Autodesk Fusion 360 part; units mm, degrees
(part 3 of 10)
  line L1783 (-29.0015, -12.4722) -> (-29.0035, -12.4576)
  line L1784 (-29.0035, -12.4576) -> (-28.9989, -12.4287)
  line L1785 (-28.9989, -12.4287) -> (-28.9835, -12.4038)
  line L1786 (-28.9835, -12.4038) -> (-28.9598, -12.3866)
  line L1787 (-28.9598, -12.3866) -> (-28.9314, -12.3799)
  line L1788 (-28.9314, -12.3799) -> (-28.9025, -12.3845)
  line L1789 (-28.9025, -12.3845) -> (-28.8776, -12.3998)
  line L1790 (-28.8776, -12.3998) -> (-28.8604, -12.4235)
  line L1791 (-28.8604, -12.4235) -> (-28.8556, -12.4374)
  line L1792 (-28.8556, -12.4374) -> (-28.6864, -13.1483)
  line L1793 (-28.6864, -13.1483) -> (-28.5725, -12.7212)
  line L1794 (-28.5725, -12.7212) -> (-28.5712, -12.7178)
  line L1795 (-28.5712, -12.7178) -> (-28.571, -12.7163)
  line L1796 (-28.571, -12.7163) -> (-28.57, -12.7146)
  line L1797 (-28.57, -12.7146) -> (-28.5673, -12.7074)
  line L1798 (-28.5673, -12.7074) -> (-28.5613, -12.6996)
  line L1799 (-28.5613, -12.6996) -> (-28.5563, -12.691)
  line L1800 (-28.5563, -12.691) -> (-28.5525, -12.6881)
  line L1801 (-28.5525, -12.6881) -> (-28.5495, -12.6842)
  line L1802 (-28.5495, -12.6842) -> (-28.541, -12.6792)
  line L1803 (-28.541, -12.6792) -> (-28.5331, -12.6732)
  line L1804 (-28.5331, -12.6732) -> (-28.5284, -12.672)
  line L1805 (-28.5284, -12.672) -> (-28.5242, -12.6695)
  line L1806 (-28.5242, -12.6695) -> (-28.5144, -12.6682)
  line L1807 (-28.5144, -12.6682) -> (-28.5048, -12.6657)
  line L1808 (-28.5048, -12.6657) -> (-28.5, -12.6663)
  line L1809 (-28.5, -12.6663) -> (-28.4952, -12.6657)
  line L1810 (-28.4952, -12.6657) -> (-28.4856, -12.6682)
  line L1811 (-28.4856, -12.6682) -> (-28.4758, -12.6695)
  line L1812 (-28.4758, -12.6695) -> (-28.4716, -12.672)
  line L1813 (-28.4716, -12.672) -> (-28.4669, -12.6732)
  line L1814 (-28.4669, -12.6732) -> (-28.459, -12.6792)
  line L1815 (-28.459, -12.6792) -> (-28.4505, -12.6842)
  line L1816 (-28.4505, -12.6842) -> (-28.4475, -12.6881)
  line L1817 (-28.4475, -12.6881) -> (-28.4437, -12.691)
  line L1818 (-28.4437, -12.691) -> (-28.4387, -12.6996)
  line L1819 (-28.4387, -12.6996) -> (-28.4327, -12.7074)
  line L1820 (-28.4327, -12.7074) -> (-28.43, -12.7146)
  line L1821 (-28.43, -12.7146) -> (-28.429, -12.7163)
  line L1822 (-28.429, -12.7163) -> (-28.4288, -12.7178)
  line L1823 (-28.4288, -12.7178) -> (-28.4275, -12.7212)
  line L1824 (-28.4275, -12.7212) -> (-28.3136, -13.1483)
  line L1825 (-28.3136, -13.1483) -> (-28.1444, -12.4374)
  line L1826 (-28.1444, -12.4374) -> (-28.1396, -12.4235)
  line L1827 (-28.1396, -12.4235) -> (-28.1224, -12.3998)
  line L1828 (-28.1224, -12.3998) -> (-28.0975, -12.3845)
  line L1829 (-28.0975, -12.3845) -> (-28.0686, -12.3799)
  line L1830 (-28.0686, -12.3799) -> (-28.0402, -12.3867)
  line L1831 (-19.702, -11.3796) -> (-19.6696, -11.412)
  line L1832 (-19.6696, -11.412) -> (-19.665, -11.435)
  line L1833 (-19.665, -11.435) -> (-19.665, -25.405)
  line L1834 (-19.665, -25.405) -> (-19.6696, -25.428)
  line L1835 (-19.6696, -25.428) -> (-19.702, -25.4604)
  line L1836 (-19.702, -25.4604) -> (-19.725, -25.465)
  line L1837 (-19.725, -25.465) -> (-33.695, -25.465)
  line L1838 (-33.695, -25.465) -> (-33.718, -25.4604)
  line L1839 (-33.718, -25.4604) -> (-33.7504, -25.428)
  line L1840 (-33.7504, -25.428) -> (-33.755, -25.405)
  line L1841 (-33.755, -25.405) -> (-33.755, -11.435)
  line L1842 (-33.755, -11.435) -> (-33.7504, -11.412)
  line L1843 (-33.7504, -11.412) -> (-33.718, -11.3796)
  line L1844 (-33.718, -11.3796) -> (-33.695, -11.375)
  line L1845 (-33.695, -11.375) -> (-19.725, -11.375)
  line L1846 (-19.725, -11.375) -> (-19.702, -11.3796)
  line L1847 (-33.635, -11.495) -> (-33.635, -25.345)
  line L1848 (-33.635, -25.345) -> (-19.785, -25.345)
  line L1849 (-19.785, -25.345) -> (-19.785, -11.495)
  line L1850 (-19.785, -11.495) -> (-33.635, -11.495)
  line L1851 (-14.3974, -12.3805) -> (-14.3954, -12.3804)
  line L1852 (-14.3954, -12.3804) -> (-14.3928, -12.381)
  line L1853 (-14.3928, -12.381) -> (-14.3901, -12.3813)
  line L1854 (-14.3901, -12.3813) -> (-14.3883, -12.382)
  line L1855 (-14.3883, -12.382) -> (-14.381, -12.3837)
  line L1856 (-14.381, -12.3837) -> (-14.2382, -12.4313)
  line L1857 (-14.2382, -12.4313) -> (-14.2248, -12.4373)
  line L1858 (-14.2248, -12.4373) -> (-14.2027, -12.4565)
  line L1859 (-14.2027, -12.4565) -> (-14.1896, -12.4826)
  line L1860 (-14.1896, -12.4826) -> (-14.1875, -12.5118)
  line L1861 (-14.1875, -12.5118) -> (-14.1967, -12.5396)
  line L1862 (-14.1967, -12.5396) -> (-14.2159, -12.5617)
  line L1863 (-14.2159, -12.5617) -> (-14.2421, -12.5748)
  line L1864 (-14.2421, -12.5748) -> (-14.2713, -12.5768)
  line L1865 (-14.2713, -12.5768) -> (-14.2856, -12.5736)
  line L1866 (-14.2856, -12.5736) -> (-14.4169, -12.5298)
  line L1867 (-14.4169, -12.5298) -> (-14.6252, -12.5298)
  line L1868 (-14.6252, -12.5298) -> (-14.6937, -12.5641)
  line L1869 (-14.6937, -12.5641) -> (-14.7241, -12.5945)
  line L1870 (-14.7241, -12.5945) -> (-14.7583, -12.663)
  line L1871 (-14.7583, -12.663) -> (-14.7583, -12.7228)
  line L1872 (-14.7583, -12.7228) -> (-14.7241, -12.7913)
  line L1873 (-14.7241, -12.7913) -> (-14.6937, -12.8218)
  line L1874 (-14.6937, -12.8218) -> (-14.6167, -12.8602)
  line L1875 (-14.6167, -12.8602) -> (-14.4342, -12.9059)
  line L1876 (-14.4342, -12.9059) -> (-14.4331, -12.9063)
  line L1877 (-14.4331, -12.9063) -> (-14.4326, -12.9063)
  line L1878 (-14.4326, -12.9063) -> (-14.4265, -12.9086)
  line L1879 (-14.4265, -12.9086) -> (-14.4203, -12.9108)
  line L1880 (-14.4203, -12.9108) -> (-14.4199, -12.9111)
  line L1881 (-14.4199, -12.9111) -> (-14.4188, -12.9115)
  line L1882 (-14.4188, -12.9115) -> (-14.3236, -12.9592)
  line L1883 (-14.3236, -12.9592) -> (-14.3173, -12.9631)
  line L1884 (-14.3173, -12.9631) -> (-14.3155, -12.9639)
  line L1885 (-14.3155, -12.9639) -> (-14.3134, -12.9656)
  line L1886 (-14.3134, -12.9656) -> (-14.3112, -12.967)
  line L1887 (-14.3112, -12.967) -> (-14.3099, -12.9685)
  line L1888 (-14.3099, -12.9685) -> (-14.3041, -12.9732)
  line L1889 (-14.3041, -12.9732) -> (-14.2565, -13.0208)
  line L1890 (-14.2565, -13.0208) -> (-14.2518, -13.0266)
  line L1891 (-14.2518, -13.0266) -> (-14.2503, -13.0279)
  line L1892 (-14.2503, -13.0279) -> (-14.2489, -13.0301)
  line L1893 (-14.2489, -13.0301) -> (-14.2472, -13.0322)
  line L1894 (-14.2472, -13.0322) -> (-14.2464, -13.034)
  line L1895 (-14.2464, -13.034) -> (-14.2424, -13.0403)
  line L1896 (-14.2424, -13.0403) -> (-14.1948, -13.1356)
  line L1897 (-14.1948, -13.1356) -> (-14.1896, -13.1493)
  line L1898 (-14.1896, -13.1493) -> (-14.1894, -13.152)
  line L1899 (-14.1894, -13.152) -> (-14.1883, -13.1545)
  line L1900 (-14.1883, -13.1545) -> (-14.1869, -13.1691)
  line L1901 (-14.1869, -13.1691) -> (-14.1869, -13.2643)
  line L1902 (-14.1869, -13.2643) -> (-14.1883, -13.279)
  line L1903 (-14.1883, -13.279) -> (-14.1894, -13.2815)
  line L1904 (-14.1894, -13.2815) -> (-14.1896, -13.2842)
  line L1905 (-14.1896, -13.2842) -> (-14.1948, -13.2979)
  line L1906 (-14.1948, -13.2979) -> (-14.2424, -13.3931)
  line L1907 (-14.2424, -13.3931) -> (-14.2464, -13.3994)
  line L1908 (-14.2464, -13.3994) -> (-14.2472, -13.4012)
  line L1909 (-14.2472, -13.4012) -> (-14.2489, -13.4033)
  line L1910 (-14.2489, -13.4033) -> (-14.2503, -13.4056)
  line L1911 (-14.2503, -13.4056) -> (-14.2518, -13.4069)
  line L1912 (-14.2518, -13.4069) -> (-14.2565, -13.4126)
  line L1913 (-14.2565, -13.4126) -> (-14.3041, -13.4602)
  line L1914 (-14.3041, -13.4602) -> (-14.3099, -13.4649)
  line L1915 (-14.3099, -13.4649) -> (-14.3112, -13.4665)
  line L1916 (-14.3112, -13.4665) -> (-14.3134, -13.4679)
  line L1917 (-14.3134, -13.4679) -> (-14.3155, -13.4696)
  line L1918 (-14.3155, -13.4696) -> (-14.3173, -13.4703)
  line L1919 (-14.3173, -13.4703) -> (-14.3236, -13.4743)
  line L1920 (-14.3236, -13.4743) -> (-14.4188, -13.5219)
  line L1921 (-14.4188, -13.5219) -> (-14.4326, -13.5272)
  line L1922 (-14.4326, -13.5272) -> (-14.4353, -13.5273)
  line L1923 (-14.4353, -13.5273) -> (-14.4377, -13.5284)
  line L1924 (-14.4377, -13.5284) -> (-14.4524, -13.5298)
  line L1925 (-14.4524, -13.5298) -> (-14.6905, -13.5298)
  line L1926 (-14.6905, -13.5298) -> (-14.6979, -13.5291)
  line L1927 (-14.6979, -13.5291) -> (-14.6999, -13.5292)
  line L1928 (-14.6999, -13.5292) -> (-14.7025, -13.5286)
  line L1929 (-14.7025, -13.5286) -> (-14.7051, -13.5284)
  line L1930 (-14.7051, -13.5284) -> (-14.7069, -13.5276)
  line L1931 (-14.7069, -13.5276) -> (-14.7142, -13.526)
  line L1932 (-14.7142, -13.526) -> (-14.857, -13.4784)
  line L1933 (-14.857, -13.4784) -> (-14.8705, -13.4724)
  line L1934 (-14.8705, -13.4724) -> (-14.8926, -13.4532)
  line L1935 (-14.8926, -13.4532) -> (-14.9057, -13.427)
  line L1936 (-14.9057, -13.427) -> (-14.9077, -13.3978)
  line L1937 (-14.9077, -13.3978) -> (-14.8985, -13.3701)
  line L1938 (-14.8985, -13.3701) -> (-14.8793, -13.3479)
  line L1939 (-14.8793, -13.3479) -> (-14.8531, -13.3349)
  line L1940 (-14.8531, -13.3349) -> (-14.824, -13.3328)
  line L1941 (-14.824, -13.3328) -> (-14.8096, -13.336)
  line L1942 (-14.8096, -13.336) -> (-14.6783, -13.3798)
  line L1943 (-14.6783, -13.3798) -> (-14.4701, -13.3798)
  line L1944 (-14.4701, -13.3798) -> (-14.4016, -13.3456)
  line L1945 (-14.4016, -13.3456) -> (-14.3712, -13.3152)
  line L1946 (-14.3712, -13.3152) -> (-14.3369, -13.2466)
  line L1947 (-14.3369, -13.2466) -> (-14.3369, -13.1868)
  line L1948 (-14.3369, -13.1868) -> (-14.3712, -13.1183)
  line L1949 (-14.3712, -13.1183) -> (-14.4016, -13.0879)
  line L1950 (-14.4016, -13.0879) -> (-14.4786, -13.0494)
  line L1951 (-14.4786, -13.0494) -> (-14.661, -13.0038)
  line L1952 (-14.661, -13.0038) -> (-14.6621, -13.0034)
  line L1953 (-14.6621, -13.0034) -> (-14.6627, -13.0033)
  line L1954 (-14.6627, -13.0033) -> (-14.6688, -13.001)
  line L1955 (-14.6688, -13.001) -> (-14.6749, -12.9988)
  line L1956 (-14.6749, -12.9988) -> (-14.6753, -12.9985)
  line L1957 (-14.6753, -12.9985) -> (-14.6764, -12.9981)
  line L1958 (-14.6764, -12.9981) -> (-14.7716, -12.9505)
  line L1959 (-14.7716, -12.9505) -> (-14.7779, -12.9465)
  line L1960 (-14.7779, -12.9465) -> (-14.7798, -12.9458)
  line L1961 (-14.7798, -12.9458) -> (-14.7818, -12.9441)
  line L1962 (-14.7818, -12.9441) -> (-14.7841, -12.9426)
  line L1963 (-14.7841, -12.9426) -> (-14.7854, -12.9411)
  line L1964 (-14.7854, -12.9411) -> (-14.7911, -12.9364)
  line L1965 (-14.7911, -12.9364) -> (-14.8387, -12.8888)
  line L1966 (-14.8387, -12.8888) -> (-14.8435, -12.8831)
  line L1967 (-14.8435, -12.8831) -> (-14.845, -12.8818)
  line L1968 (-14.845, -12.8818) -> (-14.8464, -12.8795)
  line L1969 (-14.8464, -12.8795) -> (-14.8481, -12.8774)
  line L1970 (-14.8481, -12.8774) -> (-14.8488, -12.8756)
  line L1971 (-14.8488, -12.8756) -> (-14.8528, -12.8693)
  line L1972 (-14.8528, -12.8693) -> (-14.9004, -12.7741)
  line L1973 (-14.9004, -12.7741) -> (-14.9057, -12.7603)
  line L1974 (-14.9057, -12.7603) -> (-14.9059, -12.7577)
  line L1975 (-14.9059, -12.7577) -> (-14.9069, -12.7552)
  line L1976 (-14.9069, -12.7552) -> (-14.9083, -12.7405)
  line L1977 (-14.9083, -12.7405) -> (-14.9083, -12.6453)
  line L1978 (-14.9083, -12.6453) -> (-14.9069, -12.6307)
  line L1979 (-14.9069, -12.6307) -> (-14.9059, -12.6282)
  line L1980 (-14.9059, -12.6282) -> (-14.9057, -12.6255)
  line L1981 (-14.9057, -12.6255) -> (-14.9004, -12.6118)
  line L1982 (-14.9004, -12.6118) -> (-14.8528, -12.5165)
  line L1983 (-14.8528, -12.5165) -> (-14.8488, -12.5102)
  line L1984 (-14.8488, -12.5102) -> (-14.8481, -12.5084)
  line L1985 (-14.8481, -12.5084) -> (-14.8464, -12.5063)
  line L1986 (-14.8464, -12.5063) -> (-14.845, -12.5041)
  line L1987 (-14.845, -12.5041) -> (-14.8435, -12.5028)
  line L1988 (-14.8435, -12.5028) -> (-14.8387, -12.497)
  line L1989 (-14.8387, -12.497) -> (-14.7911, -12.4494)
  line L1990 (-14.7911, -12.4494) -> (-14.7854, -12.4447)
  line L1991 (-14.7854, -12.4447) -> (-14.7841, -12.4432)
  line L1992 (-14.7841, -12.4432) -> (-14.7818, -12.4418)
  line L1993 (-14.7818, -12.4418) -> (-14.7798, -12.4401)
  line L1994 (-14.7798, -12.4401) -> (-14.7779, -12.4393)
  line L1995 (-14.7779, -12.4393) -> (-14.7716, -12.4354)
  line L1996 (-14.7716, -12.4354) -> (-14.6764, -12.3877)
  line L1997 (-14.6764, -12.3877) -> (-14.6627, -12.3825)
  line L1998 (-14.6627, -12.3825) -> (-14.66, -12.3823)
  line L1999 (-14.66, -12.3823) -> (-14.6575, -12.3813)
  line L2000 (-14.6575, -12.3813) -> (-14.6429, -12.3798)
  line L2001 (-14.6429, -12.3798) -> (-14.4048, -12.3798)
  line L2002 (-14.4048, -12.3798) -> (-14.3974, -12.3805)
  line L2003 (-12.2473, -12.3813) -> (-12.2202, -12.3925)
  line L2004 (-12.2202, -12.3925) -> (-12.1995, -12.4132)
  line L2005 (-12.1995, -12.4132) -> (-12.1883, -12.4402)
  line L2006 (-12.1883, -12.4402) -> (-12.1883, -12.4695)
  line L2007 (-12.1883, -12.4695) -> (-12.1995, -12.4965)
  line L2008 (-12.1995, -12.4965) -> (-12.2202, -12.5172)
  line L2009 (-12.2202, -12.5172) -> (-12.2473, -12.5284)
  line L2010 (-12.2473, -12.5284) -> (-12.2619, -12.5298)
  line L2011 (-12.2619, -12.5298) -> (-12.4347, -12.5298)
  line L2012 (-12.4347, -12.5298) -> (-12.5032, -12.5641)
  line L2013 (-12.5032, -12.5641) -> (-12.537, -12.5978)
  line L2014 (-12.537, -12.5978) -> (-12.6209, -12.7237)
  line L2015 (-12.6209, -12.7237) -> (-12.6394, -12.7978)
  line L2016 (-12.6394, -12.7978) -> (-12.5812, -12.7687)
  line L2017 (-12.5812, -12.7687) -> (-12.5674, -12.7634)
  line L2018 (-12.5674, -12.7634) -> (-12.5647, -12.7632)
  line L2019 (-12.5647, -12.7632) -> (-12.5623, -12.7622)
  line L2020 (-12.5623, -12.7622) -> (-12.5476, -12.7608)
  line L2021 (-12.5476, -12.7608) -> (-12.3571, -12.7608)
  line L2022 (-12.3571, -12.7608) -> (-12.3425, -12.7622)
  line L2023 (-12.3425, -12.7622) -> (-12.34, -12.7632)
  line L2024 (-12.34, -12.7632) -> (-12.3373, -12.7634)
  line L2025 (-12.3373, -12.7634) -> (-12.3236, -12.7687)
  line L2026 (-12.3236, -12.7687) -> (-12.2284, -12.8163)
  line L2027 (-12.2284, -12.8163) -> (-12.2221, -12.8203)
  line L2028 (-12.2221, -12.8203) -> (-12.2202, -12.821)
  line L2029 (-12.2202, -12.821) -> (-12.2182, -12.8227)
  line L2030 (-12.2182, -12.8227) -> (-12.2159, -12.8241)
  line L2031 (-12.2159, -12.8241) -> (-12.2146, -12.8256)
  line L2032 (-12.2146, -12.8256) -> (-12.2089, -12.8304)
  line L2033 (-12.2089, -12.8304) -> (-12.1613, -12.878)
  line L2034 (-12.1613, -12.878) -> (-12.1565, -12.8837)
  line L2035 (-12.1565, -12.8837) -> (-12.155, -12.885)
  line L2036 (-12.155, -12.885) -> (-12.1536, -12.8873)
  line L2037 (-12.1536, -12.8873) -> (-12.1519, -12.8893)
  line L2038 (-12.1519, -12.8893) -> (-12.1512, -12.8912)
  line L2039 (-12.1512, -12.8912) -> (-12.1472, -12.8975)
  line L2040 (-12.1472, -12.8975) -> (-12.0996, -12.9927)
  line L2041 (-12.0996, -12.9927) -> (-12.0943, -13.0064)
  line L2042 (-12.0943, -13.0064) -> (-12.0941, -13.0091)
  line L2043 (-12.0941, -13.0091) -> (-12.0931, -13.0116)
  line L2044 (-12.0931, -13.0116) -> (-12.0917, -13.0262)
  line L2045 (-12.0917, -13.0262) -> (-12.0917, -13.2643)
  line L2046 (-12.0917, -13.2643) -> (-12.0931, -13.279)
  line L2047 (-12.0931, -13.279) -> (-12.0941, -13.2815)
  line L2048 (-12.0941, -13.2815) -> (-12.0943, -13.2842)
  line L2049 (-12.0943, -13.2842) -> (-12.0996, -13.2979)
  line L2050 (-12.0996, -13.2979) -> (-12.1472, -13.3931)
  line L2051 (-12.1472, -13.3931) -> (-12.1512, -13.3994)
  line L2052 (-12.1512, -13.3994) -> (-12.1519, -13.4012)
  line L2053 (-12.1519, -13.4012) -> (-12.1536, -13.4033)
  line L2054 (-12.1536, -13.4033) -> (-12.155, -13.4056)
  line L2055 (-12.155, -13.4056) -> (-12.1565, -13.4069)
  line L2056 (-12.1565, -13.4069) -> (-12.1613, -13.4126)
  line L2057 (-12.1613, -13.4126) -> (-12.2089, -13.4602)
  line L2058 (-12.2089, -13.4602) -> (-12.2146, -13.4649)
  line L2059 (-12.2146, -13.4649) -> (-12.2159, -13.4665)
  line L2060 (-12.2159, -13.4665) -> (-12.2182, -13.4679)
  line L2061 (-12.2182, -13.4679) -> (-12.2202, -13.4696)
  line L2062 (-12.2202, -13.4696) -> (-12.2221, -13.4703)
  line L2063 (-12.2221, -13.4703) -> (-12.2284, -13.4743)
  line L2064 (-12.2284, -13.4743) -> (-12.3236, -13.5219)
  line L2065 (-12.3236, -13.5219) -> (-12.3373, -13.5272)
  line L2066 (-12.3373, -13.5272) -> (-12.34, -13.5273)
  line L2067 (-12.34, -13.5273) -> (-12.3425, -13.5284)
  line L2068 (-12.3425, -13.5284) -> (-12.3571, -13.5298)
  line L2069 (-12.3571, -13.5298) -> (-12.5476, -13.5298)
  line L2070 (-12.5476, -13.5298) -> (-12.5623, -13.5284)
  line L2071 (-12.5623, -13.5284) -> (-12.5647, -13.5273)
  line L2072 (-12.5647, -13.5273) -> (-12.5674, -13.5272)
  line L2073 (-12.5674, -13.5272) -> (-12.5812, -13.5219)
  line L2074 (-12.5812, -13.5219) -> (-12.6764, -13.4743)
  line L2075 (-12.6764, -13.4743) -> (-12.6827, -13.4703)
  line L2076 (-12.6827, -13.4703) -> (-12.6845, -13.4696)
  line L2077 (-12.6845, -13.4696) -> (-12.6866, -13.4679)
  line L2078 (-12.6866, -13.4679) -> (-12.6888, -13.4665)
  line L2079 (-12.6888, -13.4665) -> (-12.6901, -13.4649)
  line L2080 (-12.6901, -13.4649) -> (-12.6959, -13.4602)
  line L2081 (-12.6959, -13.4602) -> (-12.7435, -13.4126)
  line L2082 (-12.7435, -13.4126) -> (-12.7482, -13.4069)
  line L2083 (-12.7482, -13.4069) -> (-12.7497, -13.4056)
  line L2084 (-12.7497, -13.4056) -> (-12.7511, -13.4033)
  line L2085 (-12.7511, -13.4033) -> (-12.7528, -13.4012)
  line L2086 (-12.7528, -13.4012) -> (-12.7536, -13.3994)
  line L2087 (-12.7536, -13.3994) -> (-12.7576, -13.3931)
  line L2088 (-12.7576, -13.3931) -> (-12.8052, -13.2979)
  line L2089 (-12.8052, -13.2979) -> (-12.8104, -13.2842)
  line L2090 (-12.8104, -13.2842) -> (-12.8106, -13.2815)
  line L2091 (-12.8106, -13.2815) -> (-12.8117, -13.279)
  line L2092 (-12.8117, -13.279) -> (-12.8131, -13.2643)
  line L2093 (-12.8131, -13.2643) -> (-12.8131, -12.8834)
  line L2094 (-12.8131, -12.8834) -> (-12.8128, -12.8808)
  line L2095 (-12.8128, -12.8808) -> (-12.813, -12.8797)
  line L2096 (-12.813, -12.8797) -> (-12.8122, -12.8743)
  line L2097 (-12.8122, -12.8743) -> (-12.8117, -12.8688)
  line L2098 (-12.8117, -12.8688) -> (-12.8112, -12.8677)
  line L2099 (-12.8112, -12.8677) -> (-12.8109, -12.8652)
  line L2100 (-12.8109, -12.8652) -> (-12.7632, -12.6747)
  line L2101 (-12.7632, -12.6747) -> (-12.7602, -12.6661)
  line L2102 (-12.7602, -12.6661) -> (-12.7598, -12.6643)
  line L2103 (-12.7598, -12.6643) -> (-12.7589, -12.6626)
  line L2104 (-12.7589, -12.6626) -> (-12.7583, -12.6609)
  line L2105 (-12.7583, -12.6609) -> (-12.7572, -12.6594)
  line L2106 (-12.7572, -12.6594) -> (-12.7529, -12.6513)
  line L2107 (-12.7529, -12.6513) -> (-12.6576, -12.5085)
  line L2108 (-12.6576, -12.5085) -> (-12.6576, -12.5084)
  line L2109 (-12.6576, -12.5084) -> (-12.6576, -12.5084)
  line L2110 (-12.6576, -12.5084) -> (-12.6531, -12.5029)
  line L2111 (-12.6531, -12.5029) -> (-12.6483, -12.4971)
  line L2112 (-12.6483, -12.4971) -> (-12.6483, -12.4971)
  line L2113 (-12.6483, -12.4971) -> (-12.6483, -12.497)
  line L2114 (-12.6483, -12.497) -> (-12.6007, -12.4494)
  line L2115 (-12.6007, -12.4494) -> (-12.5949, -12.4447)
  line L2116 (-12.5949, -12.4447) -> (-12.5936, -12.4432)
  line L2117 (-12.5936, -12.4432) -> (-12.5913, -12.4418)
  line L2118 (-12.5913, -12.4418) -> (-12.5893, -12.4401)
  line L2119 (-12.5893, -12.4401) -> (-12.5875, -12.4393)
  line L2120 (-12.5875, -12.4393) -> (-12.5812, -12.4354)
  line L2121 (-12.5812, -12.4354) -> (-12.4859, -12.3877)
  line L2122 (-12.4859, -12.3877) -> (-12.4722, -12.3825)
  line L2123 (-12.4722, -12.3825) -> (-12.4695, -12.3823)
  line L2124 (-12.4695, -12.3823) -> (-12.467, -12.3813)
  line L2125 (-12.467, -12.3813) -> (-12.4524, -12.3798)
  line L2126 (-12.4524, -12.3798) -> (-12.2619, -12.3798)
  line L2127 (-12.2619, -12.3798) -> (-12.2473, -12.3813)
  line L2128 (-12.5984, -12.945) -> (-12.6288, -12.9754)
  line L2129 (-12.6288, -12.9754) -> (-12.6631, -13.044)
  line L2130 (-12.6631, -13.044) -> (-12.6631, -13.2466)
  line L2131 (-12.6631, -13.2466) -> (-12.6288, -13.3152)
  line L2132 (-12.6288, -13.3152) -> (-12.5984, -13.3456)
  line L2133 (-12.5984, -13.3456) -> (-12.5299, -13.3798)
  line L2134 (-12.5299, -13.3798) -> (-12.3748, -13.3798)
  line L2135 (-12.3748, -13.3798) -> (-12.3063, -13.3456)
  line L2136 (-12.3063, -13.3456) -> (-12.2759, -13.3152)
  line L2137 (-12.2759, -13.3152) -> (-12.2417, -13.2466)
  line L2138 (-12.2417, -13.2466) -> (-12.2417, -13.044)
  line L2139 (-12.2417, -13.044) -> (-12.2759, -12.9754)
  line L2140 (-12.2759, -12.9754) -> (-12.3063, -12.945)
  line L2141 (-12.3063, -12.945) -> (-12.3748, -12.9108)
  line L2142 (-12.3748, -12.9108) -> (-12.5299, -12.9108)
  line L2143 (-12.5299, -12.9108) -> (-12.5984, -12.945)
  line L2144 (-13.0402, -12.3867) -> (-13.0164, -12.4038)
  line L2145 (-13.0164, -12.4038) -> (-13.0011, -12.4287)
  line L2146 (-13.0011, -12.4287) -> (-12.9965, -12.4576)
  line L2147 (-12.9965, -12.4576) -> (-12.9985, -12.4722)
  line L2148 (-12.9985, -12.4722) -> (-13.2366, -13.4722)
  line L2149 (-13.2366, -13.4722) -> (-13.2383, -13.4772)
  line L2150 (-13.2383, -13.4772) -> (-13.2385, -13.479)
  line L2151 (-13.2385, -13.479) -> (-13.2395, -13.4806)
  line L2152 (-13.2395, -13.4806) -> (-13.2414, -13.4861)
  line L2153 (-13.2414, -13.4861) -> (-13.2477, -13.4949)
  line L2154 (-13.2477, -13.4949) -> (-13.2532, -13.5043)
  line L2155 (-13.2532, -13.5043) -> (-13.2563, -13.5067)
  line L2156 (-13.2563, -13.5067) -> (-13.2585, -13.5098)
  line L2157 (-13.2585, -13.5098) -> (-13.2678, -13.5155)
  line L2158 (-13.2678, -13.5155) -> (-13.2764, -13.5221)
  line L2159 (-13.2764, -13.5221) -> (-13.2802, -13.5231)
  line L2160 (-13.2802, -13.5231) -> (-13.2834, -13.5251)
  line L2161 (-13.2834, -13.5251) -> (-13.2942, -13.5269)
  line L2162 (-13.2942, -13.5269) -> (-13.3047, -13.5297)
  line L2163 (-13.3047, -13.5297) -> (-13.3085, -13.5292)
  line L2164 (-13.3085, -13.5292) -> (-13.3123, -13.5298)
  line L2165 (-13.3123, -13.5298) -> (-13.3229, -13.5272)
  line L2166 (-13.3229, -13.5272) -> (-13.3337, -13.5258)
  line L2167 (-13.3337, -13.5258) -> (-13.337, -13.5239)
  line L2168 (-13.337, -13.5239) -> (-13.3408, -13.523)
  line L2169 (-13.3408, -13.523) -> (-13.3496, -13.5166)
  line L2170 (-13.3496, -13.5166) -> (-13.359, -13.5111)
  line L2171 (-13.359, -13.5111) -> (-13.3614, -13.5081)
  line L2172 (-13.3614, -13.5081) -> (-13.3645, -13.5058)
  line L2173 (-13.3645, -13.5058) -> (-13.3702, -13.4966)
  line L2174 (-13.3702, -13.4966) -> (-13.3768, -13.4879)
  line L2175 (-13.3768, -13.4879) -> (-13.3789, -13.4825)
  line L2176 (-13.3789, -13.4825) -> (-13.3798, -13.4809)
  line L2177 (-13.3798, -13.4809) -> (-13.3801, -13.4791)
  line L2178 (-13.3801, -13.4791) -> (-13.382, -13.4741)
  line L2179 (-13.382, -13.4741) -> (-13.5, -13.0316)
  line L2180 (-13.5, -13.0316) -> (-13.618, -13.4741)
  line L2181 (-13.618, -13.4741) -> (-13.6199, -13.4791)
  line L2182 (-13.6199, -13.4791) -> (-13.6202, -13.4809)
  line L2183 (-13.6202, -13.4809) -> (-13.6211, -13.4825)
  line L2184 (-13.6211, -13.4825) -> (-13.6232, -13.4879)
  line L2185 (-13.6232, -13.4879) -> (-13.6298, -13.4966)
  line L2186 (-13.6298, -13.4966) -> (-13.6355, -13.5058)
  line L2187 (-13.6355, -13.5058) -> (-13.6386, -13.5081)
  line L2188 (-13.6386, -13.5081) -> (-13.641, -13.5111)
  line L2189 (-13.641, -13.5111) -> (-13.6504, -13.5166)
  line L2190 (-13.6504, -13.5166) -> (-13.6592, -13.523)
  line L2191 (-13.6592, -13.523) -> (-13.663, -13.5239)
  line L2192 (-13.663, -13.5239) -> (-13.6663, -13.5258)
  line L2193 (-13.6663, -13.5258) -> (-13.6771, -13.5272)
  line L2194 (-13.6771, -13.5272) -> (-13.6877, -13.5298)
  line L2195 (-13.6877, -13.5298) -> (-13.6915, -13.5292)
  line L2196 (-13.6915, -13.5292) -> (-13.6953, -13.5297)
  line L2197 (-13.6953, -13.5297) -> (-13.7058, -13.5269)
  line L2198 (-13.7058, -13.5269) -> (-13.7166, -13.5251)
  line L2199 (-13.7166, -13.5251) -> (-13.7198, -13.5231)
  line L2200 (-13.7198, -13.5231) -> (-13.7236, -13.5221)
  line L2201 (-13.7236, -13.5221) -> (-13.7322, -13.5155)
  line L2202 (-13.7322, -13.5155) -> (-13.7415, -13.5098)
  line L2203 (-13.7415, -13.5098) -> (-13.7437, -13.5067)
  line L2204 (-13.7437, -13.5067) -> (-13.7468, -13.5043)
  line L2205 (-13.7468, -13.5043) -> (-13.7523, -13.4949)
  line L2206 (-13.7523, -13.4949) -> (-13.7586, -13.4861)
  line L2207 (-13.7586, -13.4861) -> (-13.7605, -13.4806)
  line L2208 (-13.7605, -13.4806) -> (-13.7615, -13.479)
  line L2209 (-13.7615, -13.479) -> (-13.7617, -13.4772)
  line L2210 (-13.7617, -13.4772) -> (-13.7634, -13.4722)
  line L2211 (-13.7634, -13.4722) -> (-14.0015, -12.4722)
  line L2212 (-14.0015, -12.4722) -> (-14.0035, -12.4576)
  line L2213 (-14.0035, -12.4576) -> (-13.9989, -12.4287)
  line L2214 (-13.9989, -12.4287) -> (-13.9835, -12.4038)
  line L2215 (-13.9835, -12.4038) -> (-13.9598, -12.3866)
  line L2216 (-13.9598, -12.3866) -> (-13.9314, -12.3799)
  line L2217 (-13.9314, -12.3799) -> (-13.9025, -12.3845)
  line L2218 (-13.9025, -12.3845) -> (-13.8776, -12.3998)
  line L2219 (-13.8776, -12.3998) -> (-13.8604, -12.4235)
  line L2220 (-13.8604, -12.4235) -> (-13.8556, -12.4374)
  line L2221 (-13.8556, -12.4374) -> (-13.6864, -13.1483)
  line L2222 (-13.6864, -13.1483) -> (-13.5725, -12.7212)
  line L2223 (-13.5725, -12.7212) -> (-13.5712, -12.7178)
  line L2224 (-13.5712, -12.7178) -> (-13.571, -12.7163)
  line L2225 (-13.571, -12.7163) -> (-13.57, -12.7146)
  line L2226 (-13.57, -12.7146) -> (-13.5673, -12.7074)
  line L2227 (-13.5673, -12.7074) -> (-13.5613, -12.6996)
  line L2228 (-13.5613, -12.6996) -> (-13.5563, -12.691)
  line L2229 (-13.5563, -12.691) -> (-13.5525, -12.6881)
  line L2230 (-13.5525, -12.6881) -> (-13.5495, -12.6842)
  line L2231 (-13.5495, -12.6842) -> (-13.541, -12.6792)
  line L2232 (-13.541, -12.6792) -> (-13.5331, -12.6732)
  line L2233 (-13.5331, -12.6732) -> (-13.5284, -12.672)
  line L2234 (-13.5284, -12.672) -> (-13.5242, -12.6695)
  line L2235 (-13.5242, -12.6695) -> (-13.5144, -12.6682)
  line L2236 (-13.5144, -12.6682) -> (-13.5048, -12.6657)
  line L2237 (-13.5048, -12.6657) -> (-13.5, -12.6663)
  line L2238 (-13.5, -12.6663) -> (-13.4952, -12.6657)
  line L2239 (-13.4952, -12.6657) -> (-13.4856, -12.6682)
  line L2240 (-13.4856, -12.6682) -> (-13.4758, -12.6695)
  line L2241 (-13.4758, -12.6695) -> (-13.4716, -12.672)
  line L2242 (-13.4716, -12.672) -> (-13.4669, -12.6732)
  line L2243 (-13.4669, -12.6732) -> (-13.459, -12.6792)
  line L2244 (-13.459, -12.6792) -> (-13.4505, -12.6842)
  line L2245 (-13.4505, -12.6842) -> (-13.4475, -12.6881)
  line L2246 (-13.4475, -12.6881) -> (-13.4437, -12.691)
  line L2247 (-13.4437, -12.691) -> (-13.4387, -12.6996)
  line L2248 (-13.4387, -12.6996) -> (-13.4327, -12.7074)
  line L2249 (-13.4327, -12.7074) -> (-13.43, -12.7146)
  line L2250 (-13.43, -12.7146) -> (-13.429, -12.7163)
  line L2251 (-13.429, -12.7163) -> (-13.4288, -12.7178)
  line L2252 (-13.4288, -12.7178) -> (-13.4275, -12.7212)
  line L2253 (-13.4275, -12.7212) -> (-13.3136, -13.1483)
  line L2254 (-13.3136, -13.1483) -> (-13.1444, -12.4374)
  line L2255 (-13.1444, -12.4374) -> (-13.1396, -12.4235)
  line L2256 (-13.1396, -12.4235) -> (-13.1224, -12.3998)
  line L2257 (-13.1224, -12.3998) -> (-13.0975, -12.3845)
  line L2258 (-13.0975, -12.3845) -> (-13.0686, -12.3799)
  line L2259 (-13.0686, -12.3799) -> (-13.0402, -12.3867)
  line L2260 (-4.612, -11.3796) -> (-4.5796, -11.412)
  line L2261 (-4.5796, -11.412) -> (-4.575, -11.435)
  line L2262 (-4.575, -11.435) -> (-4.575, -25.405)
  line L2263 (-4.575, -25.405) -> (-4.5796, -25.428)
  line L2264 (-4.5796, -25.428) -> (-4.612, -25.4604)
  line L2265 (-4.612, -25.4604) -> (-4.635, -25.465)
  line L2266 (-4.635, -25.465) -> (-18.605, -25.465)
  line L2267 (-18.605, -25.465) -> (-18.628, -25.4604)
  line L2268 (-18.628, -25.4604) -> (-18.6604, -25.428)
  line L2269 (-18.6604, -25.428) -> (-18.665, -25.405)
  line L2270 (-18.665, -25.405) -> (-18.665, -11.435)
  line L2271 (-18.665, -11.435) -> (-18.6604, -11.412)
  line L2272 (-18.6604, -11.412) -> (-18.628, -11.3796)
  line L2273 (-18.628, -11.3796) -> (-18.605, -11.375)
  line L2274 (-18.605, -11.375) -> (-4.635, -11.375)
  line L2275 (-4.635, -11.375) -> (-4.612, -11.3796)
  line L2276 (-18.545, -11.495) -> (-18.545, -25.345)
  line L2277 (-18.545, -25.345) -> (-4.695, -25.345)
  line L2278 (-4.695, -25.345) -> (-4.695, -11.495)
  line L2279 (-4.695, -11.495) -> (-18.545, -11.495)
  line L2280 (-29.3735, 8.6195) -> (-29.3716, 8.6196)
  line L2281 (-29.3716, 8.6196) -> (-29.369, 8.619)
  line L2282 (-29.369, 8.619) -> (-29.3663, 8.6187)
  line L2283 (-29.3663, 8.6187) -> (-29.3645, 8.618)
  line L2284 (-29.3645, 8.618) -> (-29.3572, 8.6163)
  line L2285 (-29.3572, 8.6163) -> (-29.2144, 8.5687)
  line L2286 (-29.2144, 8.5687) -> (-29.201, 8.5627)
  line L2287 (-29.201, 8.5627) -> (-29.1788, 8.5435)
  line L2288 (-29.1788, 8.5435) -> (-29.1658, 8.5174)
  line L2289 (-29.1658, 8.5174) -> (-29.1637, 8.4882)
  line L2290 (-29.1637, 8.4882) -> (-29.1729, 8.4604)
  line L2291 (-29.1729, 8.4604) -> (-29.1921, 8.4383)
  line L2292 (-29.1921, 8.4383) -> (-29.2183, 8.4252)
  line L2293 (-29.2183, 8.4252) -> (-29.2475, 8.4232)
  line L2294 (-29.2475, 8.4232) -> (-29.2618, 8.4264)
  line L2295 (-29.2618, 8.4264) -> (-29.3931, 8.4702)
  line L2296 (-29.3931, 8.4702) -> (-29.6013, 8.4702)
  line L2297 (-29.6013, 8.4702) -> (-29.6699, 8.4359)
  line L2298 (-29.6699, 8.4359) -> (-29.7003, 8.4055)
  line L2299 (-29.7003, 8.4055) -> (-29.7345, 8.337)
  line L2300 (-29.7345, 8.337) -> (-29.7345, 8.2772)
  line L2301 (-29.7345, 8.2772) -> (-29.7003, 8.2087)
  line L2302 (-29.7003, 8.2087) -> (-29.6699, 8.1782)
  line L2303 (-29.6699, 8.1782) -> (-29.5929, 8.1398)
  line L2304 (-29.5929, 8.1398) -> (-29.4104, 8.0941)
  line L2305 (-29.4104, 8.0941) -> (-29.4093, 8.0937)
  line L2306 (-29.4093, 8.0937) -> (-29.4088, 8.0937)
  line L2307 (-29.4088, 8.0937) -> (-29.4027, 8.0914)
  line L2308 (-29.4027, 8.0914) -> (-29.3965, 8.0892)
  line L2309 (-29.3965, 8.0892) -> (-29.3961, 8.0889)
  line L2310 (-29.3961, 8.0889) -> (-29.395, 8.0885)
  line L2311 (-29.395, 8.0885) -> (-29.2998, 8.0408)
  line L2312 (-29.2998, 8.0408) -> (-29.2935, 8.0369)
  line L2313 (-29.2935, 8.0369) -> (-29.2917, 8.0361)
  line L2314 (-29.2917, 8.0361) -> (-29.2896, 8.0344)
  line L2315 (-29.2896, 8.0344) -> (-29.2873, 8.033)
  line L2316 (-29.2873, 8.033) -> (-29.2861, 8.0315)
  line L2317 (-29.2861, 8.0315) -> (-29.2803, 8.0268)
  line L2318 (-29.2803, 8.0268) -> (-29.2327, 7.9792)
  line L2319 (-29.2327, 7.9792) -> (-29.228, 7.9734)
  line L2320 (-29.228, 7.9734) -> (-29.2265, 7.9721)
  line L2321 (-29.2265, 7.9721) -> (-29.225, 7.9699)
  line L2322 (-29.225, 7.9699) -> (-29.2234, 7.9678)
  line L2323 (-29.2234, 7.9678) -> (-29.2226, 7.966)
  line L2324 (-29.2226, 7.966) -> (-29.2186, 7.9597)
  line L2325 (-29.2186, 7.9597) -> (-29.171, 7.8644)
  line L2326 (-29.171, 7.8644) -> (-29.1658, 7.8507)
  line L2327 (-29.1658, 7.8507) -> (-29.1656, 7.848)
  line L2328 (-29.1656, 7.848) -> (-29.1645, 7.8455)
  line L2329 (-29.1645, 7.8455) -> (-29.1631, 7.8309)
  line L2330 (-29.1631, 7.8309) -> (-29.1631, 7.7357)
  line L2331 (-29.1631, 7.7357) -> (-29.1645, 7.721)
  line L2332 (-29.1645, 7.721) -> (-29.1656, 7.7185)
  line L2333 (-29.1656, 7.7185) -> (-29.1658, 7.7158)
  line L2334 (-29.1658, 7.7158) -> (-29.171, 7.7021)
  line L2335 (-29.171, 7.7021) -> (-29.2186, 7.6069)
  line L2336 (-29.2186, 7.6069) -> (-29.2226, 7.6006)
  line L2337 (-29.2226, 7.6006) -> (-29.2234, 7.5988)
  line L2338 (-29.2234, 7.5988) -> (-29.225, 7.5967)
  line L2339 (-29.225, 7.5967) -> (-29.2265, 7.5944)
  line L2340 (-29.2265, 7.5944) -> (-29.228, 7.5931)
  line L2341 (-29.228, 7.5931) -> (-29.2327, 7.5874)
  line L2342 (-29.2327, 7.5874) -> (-29.2803, 7.5398)
  line L2343 (-29.2803, 7.5398) -> (-29.286, 7.535)
  line L2344 (-29.286, 7.535) -> (-29.2873, 7.5335)
  line L2345 (-29.2873, 7.5335) -> (-29.2896, 7.5321)
  line L2346 (-29.2896, 7.5321) -> (-29.2917, 7.5304)
  line L2347 (-29.2917, 7.5304) -> (-29.2935, 7.5297)
  line L2348 (-29.2935, 7.5297) -> (-29.2998, 7.5257)
  line L2349 (-29.2998, 7.5257) -> (-29.395, 7.4781)
  line L2350 (-29.395, 7.4781) -> (-29.4088, 7.4728)
  line L2351 (-29.4088, 7.4728) -> (-29.4115, 7.4727)
  line L2352 (-29.4115, 7.4727) -> (-29.4139, 7.4716)
  line L2353 (-29.4139, 7.4716) -> (-29.4286, 7.4702)
  line L2354 (-29.4286, 7.4702) -> (-29.6667, 7.4702)
  line L2355 (-29.6667, 7.4702) -> (-29.6741, 7.4709)
  line L2356 (-29.6741, 7.4709) -> (-29.676, 7.4708)
  line L2357 (-29.676, 7.4708) -> (-29.6786, 7.4714)
  line L2358 (-29.6786, 7.4714) -> (-29.6813, 7.4716)
  line L2359 (-29.6813, 7.4716) -> (-29.6831, 7.4724)
  line L2360 (-29.6831, 7.4724) -> (-29.6904, 7.474)
  line L2361 (-29.6904, 7.474) -> (-29.8332, 7.5216)
  line L2362 (-29.8332, 7.5216) -> (-29.8467, 7.5276)
  line L2363 (-29.8467, 7.5276) -> (-29.8688, 7.5468)
  line L2364 (-29.8688, 7.5468) -> (-29.8819, 7.573)
  line L2365 (-29.8819, 7.573) -> (-29.8839, 7.6022)
  line L2366 (-29.8839, 7.6022) -> (-29.8747, 7.6299)
  line L2367 (-29.8747, 7.6299) -> (-29.8555, 7.652)
  line L2368 (-29.8555, 7.652) -> (-29.8293, 7.6651)
  line L2369 (-29.8293, 7.6651) -> (-29.8001, 7.6672)
  line L2370 (-29.8001, 7.6672) -> (-29.7858, 7.664)
  line L2371 (-29.7858, 7.664) -> (-29.6545, 7.6202)
  line L2372 (-29.6545, 7.6202) -> (-29.4463, 7.6202)
  line L2373 (-29.4463, 7.6202) -> (-29.3778, 7.6544)
  line L2374 (-29.3778, 7.6544) -> (-29.3474, 7.6848)
  line L2375 (-29.3474, 7.6848) -> (-29.3131, 7.7534)
  line L2376 (-29.3131, 7.7534) -> (-29.3131, 7.8132)
  line L2377 (-29.3131, 7.8132) -> (-29.3474, 7.8817)
  line L2378 (-29.3474, 7.8817) -> (-29.3778, 7.9121)
  line L2379 (-29.3778, 7.9121) -> (-29.4547, 7.9506)
  line L2380 (-29.4547, 7.9506) -> (-29.6372, 7.9962)
  line L2381 (-29.6372, 7.9962) -> (-29.6383, 7.9966)
  line L2382 (-29.6383, 7.9966) -> (-29.6389, 7.9967)
  line L2383 (-29.6389, 7.9967) -> (-29.6449, 7.999)
  line L2384 (-29.6449, 7.999) -> (-29.6511, 8.0012)
  line L2385 (-29.6511, 8.0012) -> (-29.6515, 8.0015)
  line L2386 (-29.6515, 8.0015) -> (-29.6526, 8.0019)
  line L2387 (-29.6526, 8.0019) -> (-29.7478, 8.0495)
  line L2388 (-29.7478, 8.0495) -> (-29.7541, 8.0535)
  line L2389 (-29.7541, 8.0535) -> (-29.756, 8.0542)
  line L2390 (-29.756, 8.0542) -> (-29.758, 8.0559)
  line L2391 (-29.758, 8.0559) -> (-29.7603, 8.0574)
  line L2392 (-29.7603, 8.0574) -> (-29.7616, 8.0589)
  line L2393 (-29.7616, 8.0589) -> (-29.7673, 8.0636)
  line L2394 (-29.7673, 8.0636) -> (-29.8149, 8.1112)
  line L2395 (-29.8149, 8.1112) -> (-29.8197, 8.1169)
  line L2396 (-29.8197, 8.1169) -> (-29.8212, 8.1182)
  line L2397 (-29.8212, 8.1182) -> (-29.8226, 8.1205)
  line L2398 (-29.8226, 8.1205) -> (-29.8243, 8.1226)
  line L2399 (-29.8243, 8.1226) -> (-29.825, 8.1244)
  line L2400 (-29.825, 8.1244) -> (-29.829, 8.1307)
  line L2401 (-29.829, 8.1307) -> (-29.8766, 8.2259)
  line L2402 (-29.8766, 8.2259) -> (-29.8819, 8.2397)
  line L2403 (-29.8819, 8.2397) -> (-29.8821, 8.2423)
  line L2404 (-29.8821, 8.2423) -> (-29.8831, 8.2448)
  line L2405 (-29.8831, 8.2448) -> (-29.8845, 8.2595)
  line L2406 (-29.8845, 8.2595) -> (-29.8845, 8.3547)
  line L2407 (-29.8845, 8.3547) -> (-29.8831, 8.3693)
  line L2408 (-29.8831, 8.3693) -> (-29.8821, 8.3718)
  line L2409 (-29.8821, 8.3718) -> (-29.8819, 8.3745)
  line L2410 (-29.8819, 8.3745) -> (-29.8766, 8.3882)
  line L2411 (-29.8766, 8.3882) -> (-29.829, 8.4835)
  line L2412 (-29.829, 8.4835) -> (-29.825, 8.4898)
  line L2413 (-29.825, 8.4898) -> (-29.8243, 8.4916)
  line L2414 (-29.8243, 8.4916) -> (-29.8226, 8.4937)
  line L2415 (-29.8226, 8.4937) -> (-29.8212, 8.4959)
  line L2416 (-29.8212, 8.4959) -> (-29.8197, 8.4972)
  line L2417 (-29.8197, 8.4972) -> (-29.8149, 8.503)
  line L2418 (-29.8149, 8.503) -> (-29.7673, 8.5506)
  line L2419 (-29.7673, 8.5506) -> (-29.7616, 8.5553)
  line L2420 (-29.7616, 8.5553) -> (-29.7603, 8.5568)
  line L2421 (-29.7603, 8.5568) -> (-29.758, 8.5582)
  line L2422 (-29.758, 8.5582) -> (-29.756, 8.5599)
  line L2423 (-29.756, 8.5599) -> (-29.7541, 8.5607)
  line L2424 (-29.7541, 8.5607) -> (-29.7478, 8.5646)
  line L2425 (-29.7478, 8.5646) -> (-29.6526, 8.6123)
  line L2426 (-29.6526, 8.6123) -> (-29.6389, 8.6175)
  line L2427 (-29.6389, 8.6175) -> (-29.6362, 8.6177)
  line L2428 (-29.6362, 8.6177) -> (-29.6337, 8.6187)
  line L2429 (-29.6337, 8.6187) -> (-29.619, 8.6202)
  line L2430 (-29.619, 8.6202) -> (-29.381, 8.6202)
  line L2431 (-29.381, 8.6202) -> (-29.3735, 8.6195)
  line L2432 (-27.4214, 8.6187) -> (-27.4139, 8.6187)
  line L2433 (-27.4139, 8.6187) -> (-27.4072, 8.6159)
  line L2434 (-27.4072, 8.6159) -> (-27.3999, 8.6145)
  line L2435 (-27.3999, 8.6145) -> (-27.3938, 8.6104)
  line L2436 (-27.3938, 8.6104) -> (-27.3869, 8.6075)
  line L2437 (-27.3869, 8.6075) -> (-27.3817, 8.6023)
  line L2438 (-27.3817, 8.6023) -> (-27.3756, 8.5983)
  line L2439 (-27.3756, 8.5983) -> (-27.3715, 8.5921)
  line L2440 (-27.3715, 8.5921) -> (-27.3662, 8.5868)
  line L2441 (-27.3662, 8.5868) -> (-27.3634, 8.5801)
  line L2442 (-27.3634, 8.5801) -> (-27.3593, 8.574)
  line L2443 (-27.3593, 8.574) -> (-27.3579, 8.5667)
  line L2444 (-27.3579, 8.5667) -> (-27.355, 8.5598)
  line L2445 (-27.355, 8.5598) -> (-27.3536, 8.5453)
  line L2446 (-27.3536, 8.5453) -> (-27.3536, 8.5453)
  line L2447 (-27.3536, 8.5453) -> (-27.3536, 8.5452)
  line L2448 (-27.3536, 8.5452) -> (-27.3536, 8.5452)
  line L2449 (-27.3536, 8.5452) -> (-27.3536, 7.6202)
  line L2450 (-27.3536, 7.6202) -> (-27.1429, 7.6202)
  line L2451 (-27.1429, 7.6202) -> (-27.1282, 7.6187)
  line L2452 (-27.1282, 7.6187) -> (-27.1012, 7.6075)
  line L2453 (-27.1012, 7.6075) -> (-27.0805, 7.5868)
  line L2454 (-27.0805, 7.5868) -> (-27.0693, 7.5598)
  line L2455 (-27.0693, 7.5598) -> (-27.0693, 7.5305)
  line L2456 (-27.0693, 7.5305) -> (-27.0805, 7.5035)
  line L2457 (-27.0805, 7.5035) -> (-27.1012, 7.4828)
  line L2458 (-27.1012, 7.4828) -> (-27.1282, 7.4716)
  line L2459 (-27.1282, 7.4716) -> (-27.1429, 7.4702)
  line L2460 (-27.1429, 7.4702) -> (-27.7143, 7.4702)
  line L2461 (-27.7143, 7.4702) -> (-27.7289, 7.4716)
  line L2462 (-27.7289, 7.4716) -> (-27.756, 7.4828)
  line L2463 (-27.756, 7.4828) -> (-27.7766, 7.5035)
  line L2464 (-27.7766, 7.5035) -> (-27.7878, 7.5305)
  line L2465 (-27.7878, 7.5305) -> (-27.7878, 7.5598)
  line L2466 (-27.7878, 7.5598) -> (-27.7766, 7.5868)
  line L2467 (-27.7766, 7.5868) -> (-27.756, 7.6075)
  line L2468 (-27.756, 7.6075) -> (-27.7289, 7.6187)
  line L2469 (-27.7289, 7.6187) -> (-27.7143, 7.6202)
  line L2470 (-27.7143, 7.6202) -> (-27.5036, 7.6202)
  line L2471 (-27.5036, 7.6202) -> (-27.5036, 8.3165)
  line L2472 (-27.5036, 8.3165) -> (-27.566, 8.2541)
  line L2473 (-27.566, 8.2541) -> (-27.5718, 8.2493)
  line L2474 (-27.5718, 8.2493) -> (-27.5731, 8.2478)
  line L2475 (-27.5731, 8.2478) -> (-27.5753, 8.2464)
  line L2476 (-27.5753, 8.2464) -> (-27.5774, 8.2447)
  line L2477 (-27.5774, 8.2447) -> (-27.5792, 8.244)
  line L2478 (-27.5792, 8.244) -> (-27.5855, 8.24)
  line L2479 (-27.5855, 8.24) -> (-27.6807, 8.1924)
  line L2480 (-27.6807, 8.1924) -> (-27.6945, 8.1871)
  line L2481 (-27.6945, 8.1871) -> (-27.7237, 8.1851)
  line L2482 (-27.7237, 8.1851) -> (-27.7514, 8.1943)
  line L2483 (-27.7514, 8.1943) -> (-27.7735, 8.2135)
  line L2484 (-27.7735, 8.2135) -> (-27.7866, 8.2397)
  line L2485 (-27.7866, 8.2397) -> (-27.7887, 8.2688)
  line L2486 (-27.7887, 8.2688) -> (-27.7794, 8.2966)
  line L2487 (-27.7794, 8.2966) -> (-27.7603, 8.3187)
  line L2488 (-27.7603, 8.3187) -> (-27.7478, 8.3265)
  line L2489 (-27.7478, 8.3265) -> (-27.6635, 8.3687)
  line L2490 (-27.6635, 8.3687) -> (-27.5821, 8.4501)
  line L2491 (-27.5821, 8.4501) -> (-27.491, 8.5868)
  line L2492 (-27.491, 8.5868) -> (-27.4909, 8.5868)
  line L2493 (-27.4909, 8.5868) -> (-27.4909, 8.5868)
  line L2494 (-27.4909, 8.5868) -> (-27.4909, 8.5869)
  line L2495 (-27.4909, 8.5869) -> (-27.4817, 8.5982)
  line L2496 (-27.4817, 8.5982) -> (-27.4755, 8.6023)
  line L2497 (-27.4755, 8.6023) -> (-27.4702, 8.6075)
  line L2498 (-27.4702, 8.6075) -> (-27.4635, 8.6104)
  line L2499 (-27.4635, 8.6104) -> (-27.4573, 8.6144)
  line L2500 (-27.4573, 8.6144) -> (-27.4501, 8.6159)
  line L2501 (-27.4501, 8.6159) -> (-27.4432, 8.6187)
  line L2502 (-27.4432, 8.6187) -> (-27.4359, 8.6187)
  line L2503 (-27.4359, 8.6187) -> (-27.4287, 8.6202)
  line L2504 (-27.4287, 8.6202) -> (-27.4214, 8.6187)
  line L2505 (-26.3663, 8.6187) -> (-26.3638, 8.6177)
  line L2506 (-26.3638, 8.6177) -> (-26.3611, 8.6175)
  line L2507 (-26.3611, 8.6175) -> (-26.3474, 8.6123)
  line L2508 (-26.3474, 8.6123) -> (-26.2522, 8.5646)
  line L2509 (-26.2522, 8.5646) -> (-26.2459, 8.5607)
  line L2510 (-26.2459, 8.5607) -> (-26.244, 8.5599)
  line L2511 (-26.244, 8.5599) -> (-26.242, 8.5582)
  line L2512 (-26.242, 8.5582) -> (-26.2397, 8.5568)
  line L2513 (-26.2397, 8.5568) -> (-26.2384, 8.5553)
  line L2514 (-26.2384, 8.5553) -> (-26.2327, 8.5506)
  line L2515 (-26.2327, 8.5506) -> (-26.1851, 8.503)
  line L2516 (-26.1851, 8.503) -> (-26.1803, 8.4972)
  line L2517 (-26.1803, 8.4972) -> (-26.1788, 8.4959)
  line L2518 (-26.1788, 8.4959) -> (-26.1774, 8.4937)
  line L2519 (-26.1774, 8.4937) -> (-26.1757, 8.4916)
  line L2520 (-26.1757, 8.4916) -> (-26.175, 8.4898)
  line L2521 (-26.175, 8.4898) -> (-26.171, 8.4835)
  line L2522 (-26.171, 8.4835) -> (-26.1234, 8.3882)
  line L2523 (-26.1234, 8.3882) -> (-26.1181, 8.3745)
  line L2524 (-26.1181, 8.3745) -> (-26.1179, 8.3718)
  line L2525 (-26.1179, 8.3718) -> (-26.1169, 8.3693)
  line L2526 (-26.1169, 8.3693) -> (-26.1155, 8.3547)
  line L2527 (-26.1155, 8.3547) -> (-26.1155, 8.2595)
  line L2528 (-26.1155, 8.2595) -> (-26.1162, 8.2521)
  line L2529 (-26.1162, 8.2521) -> (-26.1161, 8.2501)
  line L2530 (-26.1161, 8.2501) -> (-26.1167, 8.2475)
  line L2531 (-26.1167, 8.2475) -> (-26.1169, 8.2448)
  line L2532 (-26.1169, 8.2448) -> (-26.1177, 8.243)
  line L2533 (-26.1177, 8.243) -> (-26.1193, 8.2357)
  line L2534 (-26.1193, 8.2357) -> (-26.1669, 8.0929)
  line L2535 (-26.1669, 8.0929) -> (-26.1729, 8.0795)
  line L2536 (-26.1729, 8.0795) -> (-26.1747, 8.0774)
  line L2537 (-26.1747, 8.0774) -> (-26.1757, 8.0749)
  line L2538 (-26.1757, 8.0749) -> (-26.1851, 8.0636)
  line L2539 (-26.1851, 8.0636) -> (-26.6285, 7.6202)
  line L2540 (-26.6285, 7.6202) -> (-26.1905, 7.6202)
  line L2541 (-26.1905, 7.6202) -> (-26.1758, 7.6187)
  line L2542 (-26.1758, 7.6187) -> (-26.1488, 7.6075)
  line L2543 (-26.1488, 7.6075) -> (-26.1281, 7.5868)
  line L2544 (-26.1281, 7.5868) -> (-26.1169, 7.5598)
  line L2545 (-26.1169, 7.5598) -> (-26.1169, 7.5305)
  line L2546 (-26.1169, 7.5305) -> (-26.1281, 7.5035)
  line L2547 (-26.1281, 7.5035) -> (-26.1488, 7.4828)
  line L2548 (-26.1488, 7.4828) -> (-26.1758, 7.4716)
  line L2549 (-26.1758, 7.4716) -> (-26.1905, 7.4702)
  line L2550 (-26.1905, 7.4702) -> (-26.8095, 7.4702)
  line L2551 (-26.8095, 7.4702) -> (-26.8242, 7.4716)
  line L2552 (-26.8242, 7.4716) -> (-26.8512, 7.4828)
  line L2553 (-26.8512, 7.4828) -> (-26.8719, 7.5035)
  line L2554 (-26.8719, 7.5035) -> (-26.8831, 7.5305)
  line L2555 (-26.8831, 7.5305) -> (-26.8831, 7.5598)
  line L2556 (-26.8831, 7.5598) -> (-26.8719, 7.5868)
  line L2557 (-26.8719, 7.5868) -> (-26.8626, 7.5982)
  line L2558 (-26.8626, 7.5982) -> (-26.3036, 8.1571)
  line L2559 (-26.3036, 8.1571) -> (-26.2655, 8.2716)
  line L2560 (-26.2655, 8.2716) -> (-26.2655, 8.337)
  line L2561 (-26.2655, 8.337) -> (-26.2997, 8.4055)
  line L2562 (-26.2997, 8.4055) -> (-26.3301, 8.4359)
  line L2563 (-26.3301, 8.4359) -> (-26.3987, 8.4702)
  line L2564 (-26.3987, 8.4702) -> (-26.6013, 8.4702)
  line L2565 (-26.6013, 8.4702) -> (-26.6699, 8.4359)
  line L2566 (-26.6699, 8.4359) -> (-26.7089, 8.3969)
  line L2567 (-26.7089, 8.3969) -> (-26.7202, 8.3876)
  line L2568 (-26.7202, 8.3876) -> (-26.7473, 8.3764)
  line L2569 (-26.7473, 8.3764) -> (-26.7765, 8.3764)
  line L2570 (-26.7765, 8.3764) -> (-26.8036, 8.3876)
  line L2571 (-26.8036, 8.3876) -> (-26.8243, 8.4083)
  line L2572 (-26.8243, 8.4083) -> (-26.8355, 8.4353)
  line L2573 (-26.8355, 8.4353) -> (-26.8355, 8.4646)
  line L2574 (-26.8355, 8.4646) -> (-26.8243, 8.4916)
  line L2575 (-26.8243, 8.4916) -> (-26.8149, 8.503)
  line L2576 (-26.8149, 8.503) -> (-26.7673, 8.5506)
  line L2577 (-26.7673, 8.5506) -> (-26.7616, 8.5553)
  line L2578 (-26.7616, 8.5553) -> (-26.7603, 8.5568)
  line L2579 (-26.7603, 8.5568) -> (-26.758, 8.5582)
  line L2580 (-26.758, 8.5582) -> (-26.756, 8.5599)
  line L2581 (-26.756, 8.5599) -> (-26.7541, 8.5607)
  line L2582 (-26.7541, 8.5607) -> (-26.7478, 8.5646)
  line L2583 (-26.7478, 8.5646) -> (-26.6526, 8.6123)
  line L2584 (-26.6526, 8.6123) -> (-26.6389, 8.6175)
  line L2585 (-26.6389, 8.6175) -> (-26.6362, 8.6177)
  line L2586 (-26.6362, 8.6177) -> (-26.6337, 8.6187)
  line L2587 (-26.6337, 8.6187) -> (-26.619, 8.6202)
  line L2588 (-26.619, 8.6202) -> (-26.381, 8.6202)
  line L2589 (-26.381, 8.6202) -> (-26.3663, 8.6187)
  line L2590 (-28.0163, 8.6133) -> (-27.9926, 8.5962)
  line L2591 (-27.9926, 8.5962) -> (-27.9773, 8.5713)
  line L2592 (-27.9773, 8.5713) -> (-27.9727, 8.5424)
  line L2593 (-27.9727, 8.5424) -> (-27.9747, 8.5278)
  line L2594 (-27.9747, 8.5278) -> (-28.2128, 7.5278)
  line L2595 (-28.2128, 7.5278) -> (-28.2145, 7.5228)
  line L2596 (-28.2145, 7.5228) -> (-28.2147, 7.521)
  line L2597 (-28.2147, 7.521) -> (-28.2157, 7.5194)
  line L2598 (-28.2157, 7.5194) -> (-28.2175, 7.5139)
  line L2599 (-28.2175, 7.5139) -> (-28.2239, 7.5051)
  line L2600 (-28.2239, 7.5051) -> (-28.2294, 7.4957)
  line L2601 (-28.2294, 7.4957) -> (-28.2324, 7.4933)
  line L2602 (-28.2324, 7.4933) -> (-28.2347, 7.4902)
  line L2603 (-28.2347, 7.4902) -> (-28.244, 7.4845)
  line L2604 (-28.244, 7.4845) -> (-28.2526, 7.4779)
  line L2605 (-28.2526, 7.4779) -> (-28.2563, 7.4769)
  line L2606 (-28.2563, 7.4769) -> (-28.2596, 7.4749)
  line L2607 (-28.2596, 7.4749) -> (-28.2704, 7.4731)
  line L2608 (-28.2704, 7.4731) -> (-28.2809, 7.4703)
  line L2609 (-28.2809, 7.4703) -> (-28.2847, 7.4708)
  line L2610 (-28.2847, 7.4708) -> (-28.2885, 7.4702)
  line L2611 (-28.2885, 7.4702) -> (-28.2991, 7.4728)
  line L2612 (-28.2991, 7.4728) -> (-28.3099, 7.4742)
  line L2613 (-28.3099, 7.4742) -> (-28.3132, 7.4761)
  line L2614 (-28.3132, 7.4761) -> (-28.317, 7.477)
  line L2615 (-28.317, 7.477) -> (-28.3258, 7.4834)
  line L2616 (-28.3258, 7.4834) -> (-28.3352, 7.4889)
  line L2617 (-28.3352, 7.4889) -> (-28.3376, 7.4919)
  line L2618 (-28.3376, 7.4919) -> (-28.3407, 7.4942)
  line L2619 (-28.3407, 7.4942) -> (-28.3464, 7.5034)
  line L2620 (-28.3464, 7.5034) -> (-28.353, 7.5121)
  line L2621 (-28.353, 7.5121) -> (-28.355, 7.5175)
  line L2622 (-28.355, 7.5175) -> (-28.356, 7.5191)
  line L2623 (-28.356, 7.5191) -> (-28.3563, 7.5209)
  line L2624 (-28.3563, 7.5209) -> (-28.3582, 7.5259)
  line L2625 (-28.3582, 7.5259) -> (-28.4762, 7.9684)
  line L2626 (-28.4762, 7.9684) -> (-28.5942, 7.5259)
  line L2627 (-28.5942, 7.5259) -> (-28.5961, 7.5209)
  line L2628 (-28.5961, 7.5209) -> (-28.5964, 7.5191)
  line L2629 (-28.5964, 7.5191) -> (-28.5973, 7.5175)
  line L2630 (-28.5973, 7.5175) -> (-28.5994, 7.5121)
  line L2631 (-28.5994, 7.5121) -> (-28.606, 7.5034)
  line L2632 (-28.606, 7.5034) -> (-28.6117, 7.4942)
  line L2633 (-28.6117, 7.4942) -> (-28.6148, 7.4919)
  line L2634 (-28.6148, 7.4919) -> (-28.6171, 7.4889)
  line L2635 (-28.6171, 7.4889) -> (-28.6266, 7.4834)
  line L2636 (-28.6266, 7.4834) -> (-28.6354, 7.477)
  line L2637 (-28.6354, 7.477) -> (-28.6391, 7.4761)
  line L2638 (-28.6391, 7.4761) -> (-28.6425, 7.4742)
  line L2639 (-28.6425, 7.4742) -> (-28.6533, 7.4728)
  line L2640 (-28.6533, 7.4728) -> (-28.6639, 7.4702)
  line L2641 (-28.6639, 7.4702) -> (-28.6677, 7.4708)
  line L2642 (-28.6677, 7.4708) -> (-28.6715, 7.4703)
  line L2643 (-28.6715, 7.4703) -> (-28.682, 7.4731)
  line L2644 (-28.682, 7.4731) -> (-28.6928, 7.4749)
  line L2645 (-28.6928, 7.4749) -> (-28.696, 7.4769)
  line L2646 (-28.696, 7.4769) -> (-28.6998, 7.4779)
  line L2647 (-28.6998, 7.4779) -> (-28.7084, 7.4845)
  line L2648 (-28.7084, 7.4845) -> (-28.7177, 7.4902)
  line L2649 (-28.7177, 7.4902) -> (-28.7199, 7.4933)
  line L2650 (-28.7199, 7.4933) -> (-28.723, 7.4957)
  line L2651 (-28.723, 7.4957) -> (-28.7285, 7.5051)
  line L2652 (-28.7285, 7.5051) -> (-28.7348, 7.5139)
  line L2653 (-28.7348, 7.5139) -> (-28.7367, 7.5194)
  line L2654 (-28.7367, 7.5194) -> (-28.7377, 7.521)
  line L2655 (-28.7377, 7.521) -> (-28.7379, 7.5228)
  line L2656 (-28.7379, 7.5228) -> (-28.7396, 7.5278)
  line L2657 (-28.7396, 7.5278) -> (-28.9777, 8.5278)
  line L2658 (-28.9777, 8.5278) -> (-28.9797, 8.5424)
  line L2659 (-28.9797, 8.5424) -> (-28.9751, 8.5713)
  line L2660 (-28.9751, 8.5713) -> (-28.9597, 8.5962)
  line L2661 (-28.9597, 8.5962) -> (-28.936, 8.6134)
  line L2662 (-28.936, 8.6134) -> (-28.9076, 8.6201)
  line L2663 (-28.9076, 8.6201) -> (-28.8787, 8.6155)
  line L2664 (-28.8787, 8.6155) -> (-28.8537, 8.6002)
  line L2665 (-28.8537, 8.6002) -> (-28.8366, 8.5765)
  line L2666 (-28.8366, 8.5765) -> (-28.8318, 8.5626)
  line L2667 (-28.8318, 8.5626) -> (-28.6626, 7.8517)
  line L2668 (-28.6626, 7.8517) -> (-28.5487, 8.2788)
  line L2669 (-28.5487, 8.2788) -> (-28.5474, 8.2822)
  line L2670 (-28.5474, 8.2822) -> (-28.5472, 8.2837)
  line L2671 (-28.5472, 8.2837) -> (-28.5462, 8.2854)
  line L2672 (-28.5462, 8.2854) -> (-28.5435, 8.2926)
  line L2673 (-28.5435, 8.2926) -> (-28.5375, 8.3004)
  line L2674 (-28.5375, 8.3004) -> (-28.5325, 8.309)
  line L2675 (-28.5325, 8.309) -> (-28.5287, 8.3119)
  line L2676 (-28.5287, 8.3119) -> (-28.5257, 8.3158)
  line L2677 (-28.5257, 8.3158) -> (-28.5171, 8.3208)
  line L2678 (-28.5171, 8.3208) -> (-28.5093, 8.3268)